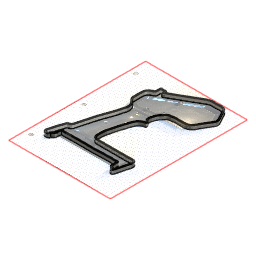
Emaxx MIrage Enclosure v0 (Autodesk Fusion 360 design; units mm, degrees)
Autodesk Fusion 360 part; units mm, degrees
sketch "Sketch2" plane through (0, 0, 0) normal (0, 0, 1) x (1, 0, 0)
  spline S0 degree 5 poles (-0.95, 3.75) (-0.9475, 3.7491) (-0.9413, 3.7486) (-0.9288, 3.7521) (-0.9057, 3.7644) (-0.869, 3.7885) (-0.8284, 3.8167) (-0.7876, 3.8442) (-0.7495, 3.8679) (-0.7146, 3.8869) (-0.6821, 3.9022) (-0.6502, 3.916) (-0.6169, 3.9306) (-0.5806, 3.948) (-0.5405, 3.9692) (-0.4968, 3.994) (-0.4504, 4.0216) (-0.4021, 4.0511) (-0.3533, 4.0811) (-0.3049, 4.1104) (-0.2575, 4.1384) (-0.2114, 4.1649) (-0.1663, 4.1901) (-0.1217, 4.2145) (-0.0769, 4.2387) (-0.0315, 4.2635) (0.0151, 4.2892) (0.0629, 4.316) (0.112, 4.3439) (0.1618, 4.3725) (0.2119, 4.4014) (0.2618, 4.43) (0.3108, 4.4579) (0.3585, 4.4847) (0.4045, 4.5102) (0.4488, 4.5344) (0.4913, 4.5578) (0.5322, 4.5804) (0.572, 4.6029) (0.6111, 4.6256) (0.6502, 4.649) (0.69, 4.6733) (0.7313, 4.6987) (0.7747, 4.7254) (0.8208, 4.7534) (0.8697, 4.7825) (0.9214, 4.8125) (0.9752, 4.8432) (1.0299, 4.8741) (1.0843, 4.9046) (1.137, 4.9344) (1.1865, 4.9628) (1.232, 4.9895) (1.2727, 5.0142) (1.3089, 5.0366) (1.3415, 5.0567) (1.3719, 5.0748) (1.4014, 5.0909) (1.4312, 5.1053) (1.4616, 5.1183) (1.4918, 5.1299) (1.5207, 5.1402) (1.5474, 5.1493) (1.5719, 5.1571) (1.5957, 5.1636) (1.6214, 5.1688) (1.6515, 5.1727) (1.6877, 5.1753) (1.7304, 5.1768) (1.7787, 5.1777) (1.831, 5.1781) (1.8853, 5.1784) (1.9398, 5.1788) (1.9928, 5.1796) (2.0435, 5.1807) (2.0916, 5.1822) (2.1375, 5.1838) (2.1815, 5.1854) (2.2245, 5.1869) (2.2669, 5.1882) (2.3091, 5.1891) (2.3512, 5.1898) (2.3932, 5.1902) (2.4348, 5.1903) (2.4757, 5.1899) (2.5154, 5.1887) (2.5536, 5.1862) (2.5898, 5.1817) (2.6236, 5.1747) (2.6548, 5.1647) (2.6834, 5.1517) (2.7093, 5.1358) (2.7329, 5.1173) (2.7545, 5.0963) (2.7746, 5.073) (2.7938, 5.047) (2.8124, 5.0181) (2.8309, 4.9862) (2.8494, 4.9516) (2.868, 4.9152) (2.8863, 4.8784) (2.9038, 4.8428) (2.9204, 4.8098) (2.9358, 4.7801) (2.9503, 4.7535) (2.9643, 4.7288) (2.9785, 4.7041) (2.9937, 4.6776) (3.0106, 4.6478) (3.0295, 4.6137) (3.0508, 4.5747) (3.0744, 4.5313) (3.0999, 4.4842) (3.1265, 4.4351) (3.1531, 4.3863) (3.1783, 4.3407) (3.2006, 4.3009) (3.2187, 4.2688) (3.2321, 4.245) (3.2409, 4.2282) (3.2464, 4.2145) (3.2505, 4.1992) (3.2546, 4.1789) (3.2598, 4.1536) (3.266, 4.1248) (3.2728, 4.0951) (3.2791, 4.0661) (3.2837, 4.0383) (3.2851, 4.0115) (3.2821, 3.985) (3.2741, 3.9576) (3.2612, 3.9283) (3.2437, 3.896) (3.2222, 3.8597) (3.1974, 3.8189) (3.1699, 3.7735) (3.1403, 3.7238) (3.109, 3.6706) (3.0764, 3.6146) (3.043, 3.5569) (3.0091, 3.4985) (2.9753, 3.4407) (2.942, 3.3841) (2.9097, 3.3298) (2.8789, 3.2782) (2.85, 3.2297) (2.8235, 3.1845) (2.7994, 3.1426) (2.7778, 3.1037) (2.7583, 3.0672) (2.7406, 3.0325) (2.7237, 2.9984) (2.7069, 2.9644) (2.6894, 2.9297) (2.6705, 2.8939) (2.6498, 2.8575) (2.627, 2.8209) (2.602, 2.785) (2.5747, 2.7507) (2.5451, 2.719) (2.5131, 2.6904) (2.4783, 2.6652) (2.4406, 2.6436) (2.3997, 2.6255) (2.3554, 2.6106) (2.3077, 2.5986) (2.2567, 2.5892) (2.2028, 2.582) (2.1464, 2.5769) (2.088, 2.5734) (2.0283, 2.5712) (1.9678, 2.5702) (1.907, 2.57) (1.8466, 2.5704) (1.7869, 2.5713) (1.7282, 2.5724) (1.6706, 2.5736) (1.6145, 2.5747) (1.5597, 2.5755) (1.5065, 2.5758) (1.4547, 2.5753) (1.4042, 2.5738) (1.355, 2.5709) (1.307, 2.5665) (1.2601, 2.5605) (1.2141, 2.5529) (1.1692, 2.5442) (1.1253, 2.5348) (1.0825, 2.5257) (1.041, 2.5175) (1.0009, 2.5106) (0.9622, 2.5051) (0.9252, 2.4999) (0.8897, 2.4934) (0.8558, 2.4834) (0.8232, 2.4678) (0.7918, 2.4453) (0.7614, 2.4157) (0.7315, 2.3802) (0.702, 2.3411) (0.6724, 2.3007) (0.6426, 2.2616) (0.6125, 2.2254) (0.5821, 2.1929) (0.5515, 2.1631) (0.5213, 2.1342) (0.4918, 2.104) (0.4634, 2.0703) (0.4367, 2.0318) (0.412, 1.9881) (0.3894, 1.9404) (0.3692, 1.8905) (0.3515, 1.8407) (0.336, 1.7932) (0.3227, 1.7498) (0.3113, 1.7112) (0.3014, 1.6772) (0.2925, 1.6462) (0.2843, 1.6167) (0.2765, 1.5869) (0.269, 1.556) (0.2617, 1.5236) (0.2552, 1.4898) (0.25, 1.4551) (0.2469, 1.4195) (0.2472, 1.3828) (0.2521, 1.3445) (0.2625, 1.3043) (0.2788, 1.2622) (0.3008, 1.2189) (0.3268, 1.1759) (0.3543, 1.1359) (0.3807, 1.1012) (0.4035, 1.074) (0.4216, 1.0551) (0.4356, 1.0436) (0.4477, 1.0366) (0.4596, 1.0305) (0.4686, 1.0229) (0.4685, 1.0131) (0.4592, 1.0035) (0.4471, 0.9978) (0.436, 0.9978) (0.4231, 1.0003) (0.4038, 1.0011) (0.3767, 0.9976) (0.3427, 0.9887) (0.3041, 0.9744) (0.2639, 0.9553) (0.2243, 0.9329) (0.1867, 0.9086) (0.1519, 0.8837) (0.1201, 0.8596) (0.0913, 0.8367) (0.065, 0.8149) (0.0406, 0.7931) (0.0175, 0.7696) (-0.0048, 0.7427) (-0.0267, 0.7112) (-0.0485, 0.6747) (-0.0701, 0.6339) (-0.0912, 0.5904) (-0.1115, 0.5459) (-0.1308, 0.5018) (-0.1487, 0.4596) (-0.1652, 0.4197) (-0.1804, 0.3815) (-0.1945, 0.3443) (-0.2078, 0.307) (-0.2206, 0.2687) (-0.233, 0.2294) (-0.2449, 0.1894) (-0.2564, 0.1499) (-0.2674, 0.112) (-0.2779, 0.0765) (-0.288, 0.0437) (-0.298, 0.0127) (-0.3085, -0.0181) (-0.3197, -0.0504) (-0.332, -0.0856) (-0.3451, -0.1237) (-0.3586, -0.1636) (-0.3717, -0.2034) (-0.3836, -0.2411) (-0.3939, -0.2749) (-0.4024, -0.3045) (-0.4097, -0.3309) (-0.4169, -0.3564) (-0.4249, -0.3836) (-0.4345, -0.4151) (-0.446, -0.4523) (-0.4593, -0.496) (-0.4738, -0.5462) (-0.4889, -0.6023) (-0.504, -0.663) (-0.5184, -0.7264) (-0.5319, -0.7901) (-0.5442, -0.8517) (-0.5555, -0.9084) (-0.566, -0.9582) (-0.5757, -0.9997) (-0.5851, -1.0326) (-0.5941, -1.0579) (-0.6028, -1.0786) (-0.6111, -1.0987) (-0.6189, -1.1217) (-0.6261, -1.1503) (-0.6329, -1.1849) (-0.6394, -1.225) (-0.6458, -1.269) (-0.6521, -1.3154) (-0.6584, -1.3628) (-0.6645, -1.4102) (-0.6701, -1.4572) (-0.6751, -1.5037) (-0.679, -1.5498) (-0.6819, -1.5956) (-0.6837, -1.6413) (-0.6844, -1.687) (-0.6843, -1.7325) (-0.6836, -1.7778) (-0.6824, -1.8227) (-0.6806, -1.8672) (-0.6778, -1.9109) (-0.6735, -1.9536) (-0.667, -1.9952) (-0.6574, -2.0354) (-0.644, -2.0738) (-0.6262, -2.1102) (-0.6039, -2.1443) (-0.577, -2.1756) (-0.5459, -2.2038) (-0.5112, -2.2287) (-0.4735, -2.2499) (-0.4341, -2.2674) (-0.3941, -2.281) (-0.3549, -2.291) (-0.3174, -2.2975) (-0.2827, -2.3011) (-0.2513, -2.3023) (-0.2231, -2.3019) (-0.1975, -2.3008) (-0.1733, -2.2996) (-0.1484, -2.2989) (-0.1198, -2.2988) (-0.0847, -2.2991) (-0.0408, -2.2998) (0.0131, -2.3004) (0.0766, -2.301) (0.1471, -2.3013) (0.2215, -2.3014) (0.2956, -2.3012) (0.3656, -2.3009) (0.428, -2.3005) (0.4805, -2.3001) (0.5223, -2.2998) (0.5549, -2.2997) (0.5819, -2.2997) (0.6078, -2.2998) (0.6374, -2.3001) (0.6744, -2.3003) (0.7211, -2.3006) (0.7787, -2.3009) (0.847, -2.3011) (0.9253, -2.3012) (1.012, -2.3011) (1.105, -2.3008) (1.2021, -2.3004) (1.3009, -2.2999) (1.3991, -2.2993) (1.4945, -2.2986) (1.5853, -2.2981) (1.6702, -2.2977) (1.748, -2.2975) (1.8179, -2.2976) (1.8797, -2.2981) (1.9336, -2.2988) (1.9802, -2.2997) (2.0208, -2.3007) (2.0572, -2.3015) (2.0915, -2.3019) (2.1261, -2.3016) (2.1628, -2.3005) (2.2031, -2.2985) (2.2474, -2.2961) (2.2952, -2.2935) (2.3455, -2.2914) (2.3967, -2.2901) (2.4466, -2.2897) (2.4931, -2.2903) (2.5337, -2.2911) (2.5664, -2.2915) (2.5903, -2.291) (2.6061, -2.2895) (2.6172, -2.2883) (2.6291, -2.2893) (2.6455, -2.2933) (2.6649, -2.2981) (2.6839, -2.3008) (2.7, -2.3016) (2.714, -2.3047) (2.728, -2.3149) (2.7429, -2.3326) (2.7584, -2.3539) (2.7733, -2.3746) (2.7863, -2.3924) (2.7959, -2.4095) (2.8013, -2.4294) (2.802, -2.4553) (2.7986, -2.4867) (2.792, -2.5219) (2.7834, -2.5581) (2.7739, -2.593) (2.7641, -2.6262) (2.7541, -2.6586) (2.7438, -2.6925) (2.7327, -2.7299) (2.7206, -2.7731) (2.7073, -2.8229) (2.6927, -2.8794) (2.6767, -2.9417) (2.6598, -3.0087) (2.642, -3.0785) (2.6237, -3.1493) (2.6056, -3.219) (2.5879, -3.2859) (2.5714, -3.3486) (2.5565, -3.4058) (2.5437, -3.4571) (2.5333, -3.502) (2.5253, -3.5406) (2.5194, -3.5732) (2.5146, -3.6005) (2.5099, -3.6233) (2.5037, -3.643) (2.4951, -3.6612) (2.4839, -3.68) (2.4709, -3.7011) (2.4573, -3.7246) (2.4445, -3.7472) (2.434, -3.7619) (2.4268, -3.762) (2.4227, -3.7469) (2.4205, -3.7222) (2.4191, -3.6951) (2.4184, -3.67) (2.4188, -3.6473) (2.4203, -3.6266) (2.4212, -3.6077) (2.4171, -3.5929) (2.4041, -3.5847) (2.3819, -3.5833) (2.3542, -3.5865) (2.3257, -3.5909) (2.3001, -3.5933) (2.2787, -3.5913) (2.2609, -3.5831) (2.2459, -3.5674) (2.2332, -3.5432) (2.2225, -3.5098) (2.2141, -3.4673) (2.2079, -3.4165) (2.2037, -3.3595) (2.2009, -3.2998) (2.1987, -3.2412) (2.1965, -3.1875) (2.1939, -3.1416) (2.1907, -3.1053) (2.1877, -3.0784) (2.1863, -3.0579) (2.1879, -3.0395) (2.1922, -3.0196) (2.1952, -2.9981) (2.1906, -2.9775) (2.1729, -2.9613) (2.1414, -2.9514) (2.1005, -2.9473) (2.0571, -2.9474) (2.0178, -2.9495) (1.987, -2.9514) (1.9639, -2.9522) (1.9434, -2.9515) (1.9189, -2.9499) (1.8844, -2.9478) (1.8365, -2.9456) (1.7739, -2.9436) (1.697, -2.9422) (1.6078, -2.9414) (1.5091, -2.9414) (1.4044, -2.9422) (1.2973, -2.9438) (1.1916, -2.9461) (1.0903, -2.9491) (0.9957, -2.9526) (0.9088, -2.9565) (0.8294, -2.9606) (0.7564, -2.9648) (0.6878, -2.9689) (0.6214, -2.9727) (0.5545, -2.9762) (0.4845, -2.9791) (0.409, -2.9815) (0.3258, -2.9832) (0.2336, -2.9843) (0.1317, -2.9847) (0.0203, -2.9845) (-0.1, -2.9839) (-0.228, -2.9829) (-0.3621, -2.9817) (-0.5004, -2.9805) (-0.6409, -2.9793) (-0.7812, -2.9783) (-0.9193, -2.9777) (-1.0531, -2.9775) (-1.1806, -2.9779) (-1.3005, -2.9788) (-1.4115, -2.9804) (-1.513, -2.9825) (-1.605, -2.9851) (-1.6882, -2.988) (-1.7639, -2.9911) (-1.8336, -2.994) (-1.8992, -2.9965) (-1.9623, -2.9986) (-2.0243, -2.9999) (-2.0862, -3.0005) (-2.1483, -3.0002) (-2.21, -2.9992) (-2.2697, -2.9977) (-2.3252, -2.9961) (-2.3741, -2.995) (-2.4146, -2.9952) (-2.4455, -2.9977) (-2.4674, -3.004) (-2.4824, -3.0159) (-2.4942, -3.0351) (-2.5057, -3.0628) (-2.5184, -3.0989) (-2.5312, -3.1418) (-2.5423, -3.1893) (-2.5496, -3.2388) (-2.5516, -3.2878) (-2.5484, -3.3344) (-2.5427, -3.3775) (-2.5391, -3.417) (-2.5424, -3.4535) (-2.5569, -3.4871) (-2.5845, -3.5182) (-2.6236, -3.546) (-2.6692, -3.5692) (-2.715, -3.5867) (-2.7546, -3.5981) (-2.7831, -3.6044) (-2.7991, -3.6085) (-2.8055, -3.616) (-2.8072, -3.6317) (-2.8077, -3.6559) (-2.8087, -3.685) (-2.8102, -3.7139) (-2.8116, -3.7385) (-2.8114, -3.7576) (-2.8096, -3.772) (-2.8089, -3.7827) (-2.8163, -3.7905) (-2.8371, -3.7957) (-2.8698, -3.7986) (-2.9085, -3.7994) (-2.946, -3.7982) (-2.9762, -3.7947) (-2.9978, -3.7883) (-3.0132, -3.7783) (-3.0259, -3.7642) (-3.0382, -3.7454) (-3.0499, -3.722) (-3.0598, -3.6944) (-3.0664, -3.6636) (-3.0689, -3.6309) (-3.0672, -3.5981) (-3.0615, -3.5667) (-3.0526, -3.5375) (-3.0414, -3.5102) (-3.029, -3.4838) (-3.0165, -3.4566) (-3.0046, -3.4272) (-2.9937, -3.3948) (-2.9837, -3.3593) (-2.9744, -3.3214) (-2.9652, -3.2818) (-2.9557, -3.2414) (-2.9456, -3.201) (-2.935, -3.1609) (-2.924, -3.1212) (-2.9129, -3.0819) (-2.9018, -3.0432) (-2.8912, -3.0051) (-2.8811, -2.9678) (-2.8718, -2.9316) (-2.863, -2.8969) (-2.8545, -2.8636) (-2.8459, -2.8317) (-2.8365, -2.8009) (-2.8256, -2.7708) (-2.8129, -2.7407) (-2.7985, -2.7105) (-2.7832, -2.6802) (-2.7687, -2.6503) (-2.7563, -2.6209) (-2.7471, -2.5923) (-2.7411, -2.5642) (-2.7373, -2.5356) (-2.7337, -2.5058) (-2.7284, -2.4744) (-2.7203, -2.4421) (-2.7087, -2.411) (-2.6938, -2.3834) (-2.676, -2.3615) (-2.6559, -2.3462) (-2.6333, -2.3362) (-2.6085, -2.3294) (-2.5813, -2.3227) (-2.5521, -2.314) (-2.5217, -2.302) (-2.4912, -2.2863) (-2.4615, -2.2667) (-2.4337, -2.2435) (-2.4086, -2.217) (-2.3867, -2.1873) (-2.3684, -2.1548) (-2.3534, -2.1198) (-2.3414, -2.0825) (-2.3316, -2.0433) (-2.323, -2.0027) (-2.3144, -1.961) (-2.3049, -1.9186) (-2.294, -1.8759) (-2.2816, -1.8329) (-2.2679, -1.7898) (-2.2538, -1.7466) (-2.2399, -1.7034) (-2.227, -1.6602) (-2.2155, -1.6171) (-2.2055, -1.5743) (-2.1966, -1.5322) (-2.1881, -1.491) (-2.1794, -1.4507) (-2.1699, -1.4113) (-2.1592, -1.3723) (-2.1471, -1.3328) (-2.1339, -1.292) (-2.1199, -1.2489) (-2.1056, -1.2029) (-2.0912, -1.1537) (-2.0774, -1.1019) (-2.0641, -1.0488) (-2.0516, -0.9961) (-2.0398, -0.9457) (-2.0287, -0.8991) (-2.0183, -0.8574) (-2.0082, -0.8208) (-1.9984, -0.7883) (-1.9887, -0.7578) (-1.9789, -0.7271) (-1.9687, -0.694) (-1.9579, -0.657) (-1.9463, -0.6154) (-1.9337, -0.5694) (-1.9199, -0.5196) (-1.9049, -0.467) (-1.8885, -0.4129) (-1.871, -0.3581) (-1.8523, -0.3036) (-1.8329, -0.2497) (-1.8131, -0.1969) (-1.7932, -0.1451) (-1.7736, -0.0945) (-1.7545, -0.0451) (-1.7363, 0.0034) (-1.7189, 0.0507) (-1.7023, 0.0971) (-1.6866, 0.1423) (-1.6714, 0.1866) (-1.6568, 0.23) (-1.6424, 0.2726) (-1.628, 0.3148) (-1.6135, 0.3569) (-1.5988, 0.3995) (-1.5837, 0.443) (-1.5683, 0.4877) (-1.5526, 0.5339) (-1.5369, 0.5816) (-1.5213, 0.6308) (-1.5062, 0.681) (-1.4919, 0.7318) (-1.4786, 0.7829) (-1.4663, 0.8335) (-1.455, 0.8832) (-1.4444, 0.9312) (-1.4341, 0.9772) (-1.4235, 1.0208) (-1.4124, 1.0616) (-1.4004, 1.0998) (-1.3877, 1.1358) (-1.3748, 1.1701) (-1.3623, 1.2038) (-1.3511, 1.2377) (-1.3418, 1.2728) (-1.335, 1.3096) (-1.3308, 1.3481) (-1.3291, 1.3884) (-1.3297, 1.4299) (-1.3323, 1.4723) (-1.3368, 1.5152) (-1.3434, 1.5582) (-1.3525, 1.6013) (-1.3643, 1.6444) (-1.3792, 1.6872) (-1.3974, 1.7296) (-1.4188, 1.7711) (-1.4428, 1.8112) (-1.4689, 1.8491) (-1.4961, 1.8842) (-1.5236, 1.9161) (-1.551, 1.9446) (-1.5778, 1.9701) (-1.6041, 1.9935) (-1.6302, 2.016) (-1.6561, 2.0386) (-1.6818, 2.0623) (-1.7069, 2.0876) (-1.7303, 2.1143) (-1.751, 2.142) (-1.7681, 2.1705) (-1.781, 2.1998) (-1.7898, 2.2305) (-1.795, 2.2636) (-1.7976, 2.2999) (-1.7984, 2.3404) (-1.7983, 2.3856) (-1.798, 2.4353) (-1.7978, 2.4889) (-1.7979, 2.5453) (-1.7984, 2.6036) (-1.7993, 2.6625) (-1.8004, 2.7209) (-1.8016, 2.7779) (-1.8027, 2.8327) (-1.8034, 2.8851) (-1.8034, 2.9347) (-1.8026, 2.9815) (-1.8005, 3.0257) (-1.7968, 3.0672) (-1.7912, 3.1064) (-1.7834, 3.1435) (-1.7729, 3.1788) (-1.7596, 3.2124) (-1.7432, 3.2445) (-1.7236, 3.2753) (-1.7008, 3.3046) (-1.675, 3.3325) (-1.6463, 3.3588) (-1.6151, 3.3836) (-1.5821, 3.4067) (-1.5478, 3.4282) (-1.513, 3.4483) (-1.4782, 3.467) (-1.4442, 3.4846) (-1.4114, 3.5015) (-1.3801, 3.5178) (-1.3507, 3.534) (-1.3238, 3.55) (-1.3004, 3.5656) (-1.2818, 3.5802) (-1.2693, 3.5933) (-1.2631, 3.6054) (-1.2618, 3.6189) (-1.2626, 3.6373) (-1.2631, 3.6633) (-1.2626, 3.698) (-1.2616, 3.7406) (-1.261, 3.7892) (-1.2616, 3.8407) (-1.2639, 3.8914) (-1.2672, 3.937) (-1.2698, 3.9733) (-1.2701, 3.9974) (-1.2665, 4.0079) (-1.2586, 4.0066) (-1.2472, 3.998) (-1.233, 3.9874) (-1.2159, 3.9784) (-1.1957, 3.973) (-1.1731, 3.9708) (-1.1494, 3.9697) (-1.1256, 3.9675) (-1.102, 3.9639) (-1.0772, 3.9617) (-1.0496, 3.9646) (-1.019, 3.9745) (-0.9883, 3.989) (-0.963, 4.0009) (-0.9481, 4.0034) (-0.9453, 3.9939) (-0.9493, 3.9789) (-0.9524, 3.9668) (-0.9517, 3.9575) (-0.9486, 3.9442) (-0.9457, 3.9222) (-0.9449, 3.8916) (-0.9473, 3.855) (-0.9527, 3.817) (-0.9584, 3.7831) (-0.9595, 3.7632) (-0.9566, 3.7542) (-0.9525, 3.7509) (-0.95, 3.75) knots 0 0 0 0 0 0 0.00123457 0.00246914 0.0037037 0.00493827 0.00617284 0.00740741 0.00864198 0.00987654 0.01111111 0.01234568 0.01358025 0.01481481 0.01604938 0.01728395 0.01851852 0.01975309 0.02098765 0.02222222 0.02345679 0.02469136 0.02592593 0.02716049 0.02839506 0.02962963 0.0308642 0.03209877 0.03333333 0.0345679 0.03580247 0.03703704 0.0382716 0.03950617 0.04074074 0.04197531 0.04320988 0.04444444 0.04567901 0.04691358 0.04814815 0.04938272 0.05061728 0.05185185 0.05308642 0.05432099 0.05555556 0.05679012 0.05802469 0.05925926 0.06049383 0.0617284 0.06296296 0.06419753 0.0654321 0.06666667 0.06790123 0.0691358 0.07037037 0.07160494 0.07283951 0.07407407 0.07530864 0.07654321 0.07777778 0.07901235 0.08024691 0.08148148 0.08271605 0.08395062 0.08518519 0.08641975 0.08765432 0.08888889 0.09012346 0.09135802 0.09259259 0.09382716 0.09506173 0.0962963 0.09753086 0.09876543 0.1 0.10123457 0.10246914 0.1037037 0.10493827 0.10617284 0.10740741 0.10864198 0.10987654 0.11111111 0.11234568 0.11358025 0.11481481 0.11604938 0.11728395 0.11851852 0.11975309 0.12098765 0.12222222 0.12345679 0.12469136 0.12592593 0.12716049 0.12839506 0.12962963 0.1308642 0.13209877 0.13333333 0.1345679 0.13580247 0.13703704 0.1382716 0.13950617 0.14074074 0.14197531 0.14320988 0.14444444 0.14567901 0.14691358 0.14814815 0.14938272 0.15061728 0.15185185 0.15308642 0.15432099 0.15555556 0.15679012 0.15802469 0.15925926 0.16049383 0.1617284 0.16296296 0.16419753 0.1654321 0.16666667 0.16790123 0.1691358 0.17037037 0.17160494 0.17283951 0.17407407 0.17530864 0.17654321 0.17777778 0.17901235 0.18024691 0.18148148 0.18271605 0.18395062 0.18518519 0.18641975 0.18765432 0.18888889 0.19012346 0.19135802 0.19259259 0.19382716 0.19506173 0.1962963 0.19753086 0.19876543 0.2 0.20123457 0.20246914 0.2037037 0.20493827 0.20617284 0.20740741 0.20864198 0.20987654 0.21111111 0.21234568 0.21358025 0.21481481 0.21604938 0.21728395 0.21851852 0.21975309 0.22098765 0.22222222 0.22345679 0.22469136 0.22592593 0.22716049 0.22839506 0.22962963 0.2308642 0.23209877 0.23333333 0.2345679 0.23580247 0.23703704 0.2382716 0.23950617 0.24074074 0.24197531 0.24320988 0.24444444 0.24567901 0.24691358 0.24814815 0.24938272 0.25061728 0.25185185 0.25308642 0.25432099 0.25555556 0.25679012 0.25802469 0.25925926 0.26049383 0.2617284 0.26296296 0.26419753 0.2654321 0.26666667 0.26790123 0.2691358 0.27037037 0.27160494 0.27283951 0.27407407 0.27530864 0.27654321 0.27777778 0.27901235 0.28024691 0.28148148 0.28271605 0.28395062 0.28518519 0.28641975 0.28765432 0.28888889 0.29012346 0.29135802 0.29259259 0.29382716 0.29506173 0.2962963 0.29753086 0.29876543 0.3 0.30123457 0.30246914 0.3037037 0.30493827 0.30617284 0.30740741 0.30864198 0.30987654 0.31111111 0.31234568 0.31358025 0.31481481 0.31604938 0.31728395 0.31851852 0.31975309 0.32098765 0.32222222 0.32345679 0.32469136 0.32592593 0.32716049 0.32839506 0.32962963 0.3308642 0.33209877 0.33333333 0.3345679 0.33580247 0.33703704 0.3382716 0.33950617 0.34074074 0.34197531 0.34320988 0.34444444 0.34567901 0.34691358 0.34814815 0.34938272 0.35061728 0.35185185 0.35308642 0.35432099 0.35555556 0.35679012 0.35802469 0.35925926 0.36049383 0.3617284 0.36296296 0.36419753 0.3654321 0.36666667 0.36790123 0.3691358 0.37037037 0.37160494 0.37283951 0.37407407 0.37530864 0.37654321 0.37777778 0.37901235 0.38024691 0.38148148 0.38271605 0.38395062 0.38518519 0.38641975 0.38765432 0.38888889 0.39012346 0.39135802 0.39259259 0.39382716 0.39506173 0.3962963 0.39753086 0.39876543 0.4 0.40123457 0.40246914 0.4037037 0.40493827 0.40617284 0.40740741 0.40864198 0.40987654 0.41111111 0.41234568 0.41358025 0.41481481 0.41604938 0.41728395 0.41851852 0.41975309 0.42098765 0.42222222 0.42345679 0.42469136 0.42592593 0.42716049 0.42839506 0.42962963 0.4308642 0.43209877 0.43333333 0.4345679 0.43580247 0.43703704 0.4382716 0.43950617 0.44074074 0.44197531 0.44320988 0.44444444 0.44567901 0.44691358 0.44814815 0.44938272 0.45061728 0.45185185 0.45308642 0.45432099 0.45555556 0.45679012 0.45802469 0.45925926 0.46049383 0.4617284 0.46296296 0.46419753 0.4654321 0.46666667 0.46790123 0.4691358 0.47037037 0.47160494 0.47283951 0.47407407 0.47530864 0.47654321 0.47777778 0.47901235 0.48024691 0.48148148 0.48271605 0.48395062 0.48518519 0.48641975 0.48765432 0.48888889 0.49012346 0.49135802 0.49259259 0.49382716 0.49506173 0.4962963 0.49753086 0.49876543 0.5 0.50123457 0.50246914 0.5037037 0.50493827 0.50617284 0.50740741 0.50864198 0.50987654 0.51111111 0.51234568 0.51358025 0.51481481 0.51604938 0.51728395 0.51851852 0.51975309 0.52098765 0.52222222 0.52345679 0.52469136 0.52592593 0.52716049 0.52839506 0.52962963 0.5308642 0.53209877 0.53333333 0.5345679 0.53580247 0.53703704 0.5382716 0.53950617 0.54074074 0.54197531 0.54320988 0.54444444 0.54567901 0.54691358 0.54814815 0.54938272 0.55061728 0.55185185 0.55308642 0.55432099 0.55555556 0.55679012 0.55802469 0.55925926 0.56049383 0.5617284 0.56296296 0.56419753 0.5654321 0.56666667 0.56790123 0.5691358 0.57037037 0.57160494 0.57283951 0.57407407 0.57530864 0.57654321 0.57777778 0.57901235 0.58024691 0.58148148 0.58271605 0.58395062 0.58518519 0.58641975 0.58765432 0.58888889 0.59012346 0.59135802 0.59259259 0.59382716 0.59506173 0.5962963 0.59753086 0.59876543 0.6 0.60123457 0.60246914 0.6037037 0.60493827 0.60617284 0.60740741 0.60864198 0.60987654 0.61111111 0.61234568 0.61358025 0.61481481 0.61604938 0.61728395 0.61851852 0.61975309 0.62098765 0.62222222 0.62345679 0.62469136 0.62592593 0.62716049 0.62839506 0.62962963 0.6308642 0.63209877 0.63333333 0.6345679 0.63580247 0.63703704 0.6382716 0.63950617 0.64074074 0.64197531 0.64320988 0.64444444 0.64567901 0.64691358 0.64814815 0.64938272 0.65061728 0.65185185 0.65308642 0.65432099 0.65555556 0.65679012 0.65802469 0.65925926 0.66049383 0.6617284 0.66296296 0.66419753 0.6654321 0.66666667 0.66790123 0.6691358 0.67037037 0.67160494 0.67283951 0.67407407 0.67530864 0.67654321 0.67777778 0.67901235 0.68024691 0.68148148 0.68271605 0.68395062 0.68518519 0.68641975 0.68765432 0.68888889 0.69012346 0.69135802 0.69259259 0.69382716 0.69506173 0.6962963 0.69753086 0.69876543 0.7 0.70123457 0.70246914 0.7037037 0.70493827 0.70617284 0.70740741 0.70864198 0.70987654 0.71111111 0.71234568 0.71358025 0.71481481 0.71604938 0.71728395 0.71851852 0.71975309 0.72098765 0.72222222 0.72345679 0.72469136 0.72592593 0.72716049 0.72839506 0.72962963 0.7308642 0.73209877 0.73333333 0.7345679 0.73580247 0.73703704 0.7382716 0.73950617 0.74074074 0.74197531 0.74320988 0.74444444 0.74567901 0.74691358 0.74814815 0.74938272 0.75061728 0.75185185 0.75308642 0.75432099 0.75555556 0.75679012 0.75802469 0.75925926 0.76049383 0.7617284 0.76296296 0.76419753 0.7654321 0.76666667 0.76790123 0.7691358 0.77037037 0.77160494 0.77283951 0.77407407 0.77530864 0.77654321 0.77777778 0.77901235 0.78024691 0.78148148 0.78271605 0.78395062 0.78518519 0.78641975 0.78765432 0.78888889 0.79012346 0.79135802 0.79259259 0.79382716 0.79506173 0.7962963 0.79753086 0.79876543 0.8 0.80123457 0.80246914 0.8037037 0.80493827 0.80617284 0.80740741 0.80864198 0.80987654 0.81111111 0.81234568 0.81358025 0.81481481 0.81604938 0.81728395 0.81851852 0.81975309 0.82098765 0.82222222 0.82345679 0.82469136 0.82592593 0.82716049 0.82839506 0.82962963 0.8308642 0.83209877 0.83333333 0.8345679 0.83580247 0.83703704 0.8382716 0.83950617 0.84074074 0.84197531 0.84320988 0.84444444 0.84567901 0.84691358 0.84814815 0.84938272 0.85061728 0.85185185 0.85308642 0.85432099 0.85555556 0.85679012 0.85802469 0.85925926 0.86049383 0.8617284 0.86296296 0.86419753 0.8654321 0.86666667 0.86790123 0.8691358 0.87037037 0.87160494 0.87283951 0.87407407 0.87530864 0.87654321 0.87777778 0.87901235 0.88024691 0.88148148 0.88271605 0.88395062 0.88518519 0.88641975 0.88765432 0.88888889 0.89012346 0.89135802 0.89259259 0.89382716 0.89506173 0.8962963 0.89753086 0.89876543 0.9 0.90123457 0.90246914 0.9037037 0.90493827 0.90617284 0.90740741 0.90864198 0.90987654 0.91111111 0.91234568 0.91358025 0.91481481 0.91604938 0.91728395 0.91851852 0.91975309 0.92098765 0.92222222 0.92345679 0.92469136 0.92592593 0.92716049 0.92839506 0.92962963 0.9308642 0.93209877 0.93333333 0.9345679 0.93580247 0.93703704 0.9382716 0.93950617 0.94074074 0.94197531 0.94320988 0.94444444 0.94567901 0.94691358 0.94814815 0.94938272 0.95061728 0.95185185 0.95308642 0.95432099 0.95555556 0.95679012 0.95802469 0.95925926 0.96049383 0.9617284 0.96296296 0.96419753 0.9654321 0.96666667 0.96790123 0.9691358 0.97037037 0.97160494 0.97283951 0.97407407 0.97530864 0.97654321 0.97777778 0.97901235 0.98024691 0.98148148 0.98271605 0.98395062 0.98518519 0.98641975 0.98765432 0.98888889 0.99012346 0.99135802 0.99259259 0.99382716 0.99506173 0.9962963 0.99753086 0.99876543 1 1 1 1 1 1
  spline S1 degree 3 poles (-1.1781, 4.0748) (-1.1778, 4.0746) (-1.1779, 4.0746) (-1.1781, 4.0748) knots 0.970853 0.970853 0.970853 0.970853 0.971274 0.971274 0.971274 0.971274
  spline S2 degree 3 poles (-0.8442, 3.9291) (-0.831, 3.9376) (-0.8196, 3.9447) (-0.8076, 3.9518) (-0.6925, 4.0201) (-0.6238, 4.0366) (-0.494, 4.1151) (-0.2507, 4.2622) (-0.0052, 4.3964) (0.2498, 4.5409) (0.4771, 4.6697) (0.6102, 4.7503) (0.8547, 4.8921) (1.0195, 4.9876) (1.1869, 5.0829) (1.2903, 5.1452) (1.3922, 5.2066) (1.4819, 5.2438) (1.5826, 5.2652) (1.7143, 5.2931) (1.9719, 5.2803) (2.1505, 5.2867) (2.3228, 5.293) (2.4851, 5.3166) (2.6506, 5.2725) (2.8553, 5.2181) (2.9472, 4.9806) (3.0181, 4.8439) (3.063, 4.7576) (3.1018, 4.6958) (3.1788, 4.5535) (3.238, 4.4442) (3.3, 4.3371) (3.3276, 4.283) (3.3619, 4.2161) (3.3764, 4.1556) (3.3855, 4.041) (3.398, 3.8843) (3.2626, 3.7314) (3.1297, 3.5024) (3.0163, 3.3067) (2.9061, 3.1292) (2.8466, 3.0146) (2.7855, 2.8971) (2.7326, 2.7484) (2.5954, 2.6273) (2.3571, 2.417) (1.9073, 2.4684) (1.5838, 2.4727) (1.3679, 2.4756) (1.2067, 2.4419) (1.0363, 2.4129) (0.9025, 2.3902) (0.8746, 2.4006) (0.7847, 2.2804) (0.7152, 2.1875) (0.6188, 2.0932) (0.5622, 2.0279) (0.482, 1.9353) (0.4248, 1.7364) (0.3949, 1.6315) (0.3655, 1.5286) (0.3307, 1.4414) (0.3586, 1.3443) (0.3758, 1.2844) (0.444, 1.1836) (0.4782, 1.1449) (0.4967, 1.1238) (0.4848, 1.1335) (0.5024, 1.1234) (0.513, 1.1174) (0.5634, 1.1007) (0.5694, 1.027) (0.5768, 0.9373) (0.5186, 0.9132) (0.4769, 0.9011) (0.425, 0.8861) (0.4162, 0.8984) (0.4082, 0.8979) (0.385, 0.8963) (0.2309, 0.8181) (0.1538, 0.7553) (0.088, 0.7017) (0.0554, 0.6595) (0.0045, 0.5526) (-0.0868, 0.3608) (-0.1391, 0.1779) (-0.1878, 0.0214) (-0.2297, -0.1128) (-0.2857, -0.2691) (-0.3163, -0.3767) (-0.3389, -0.4565) (-0.3867, -0.5992) (-0.4254, -0.7818) (-0.458, -0.936) (-0.4874, -1.0672) (-0.508, -1.1175) (-0.5249, -1.1586) (-0.5324, -1.1983) (-0.5451, -1.2891) (-0.5748, -1.5008) (-0.5919, -1.7342) (-0.5741, -1.9164) (-0.5609, -2.0511) (-0.509, -2.1258) (-0.3996, -2.1699) (-0.2973, -2.2111) (-0.2319, -2.1966) (-0.1261, -2.1965) (-0.0505, -2.1964) (0.1093, -2.1993) (0.2788, -2.1988) (0.439, -2.1984) (0.5332, -2.1971) (0.5937, -2.1974) (0.6617, -2.1977) (0.7841, -2.199) (1.0062, -2.1987) (1.3039, -2.1982) (1.6792, -2.1938) (1.8761, -2.1957) (2.079, -2.1977) (2.1306, -2.1983) (2.3057, -2.1907) (2.4079, -2.1862) (2.5287, -2.1895) (2.5715, -2.1889) (2.5974, -2.1885) (2.6142, -2.1834) (2.6474, -2.1891) (2.6891, -2.1963) (2.6669, -2.1838) (2.7389, -2.2065) (2.8053, -2.2274) (2.8328, -2.282) (2.8534, -2.3106) (2.8811, -2.3489) (2.9098, -2.4465) (2.8956, -2.5234) (2.8707, -2.6588) (2.8364, -2.7306) (2.7837, -2.9367) (2.7335, -3.1334) (2.661, -3.3989) (2.6336, -3.524) (2.6155, -3.6062) (2.6097, -3.6653) (2.5806, -3.7173) (2.5623, -3.7498) (2.5541, -3.7674) (2.5268, -3.8072) (2.5187, -3.8191) (2.5229, -3.8484) (2.4486, -3.861) (2.3957, -3.87) (2.3434, -3.8205) (2.3336, -3.7996) (2.3055, -3.7398) (2.3186, -3.7331) (2.3175, -3.7101) (2.3172, -3.7047) (2.317, -3.7) (2.3168, -3.6941) knots 0.00616262 0.00616262 0.00616262 0.00616262 0.00723627 0.00723627 0.00723627 0.01751679 0.01751679 0.01751679 0.03677766 0.03677766 0.03677766 0.05394591 0.05394591 0.05394591 0.0655192 0.0655192 0.0655192 0.07691737 0.07691737 0.07691737 0.09183359 0.09183359 0.09183359 0.10622417 0.10622417 0.10622417 0.12401706 0.12401706 0.12401706 0.13525578 0.13525578 0.13525578 0.14388411 0.14388411 0.14388411 0.15457935 0.15457935 0.15457935 0.1691993 0.1691993 0.1691993 0.1816861 0.1816861 0.1816861 0.19448952 0.19448952 0.19448952 0.21671489 0.21671489 0.21671489 0.23154272 0.23154272 0.23154272 0.24318105 0.24318105 0.24318105 0.25216346 0.25216346 0.25216346 0.26491111 0.26491111 0.26491111 0.27740929 0.27740929 0.27740929 0.28512377 0.28512377 0.28512377 0.28932444 0.28932444 0.28932444 0.29185971 0.29185971 0.29185971 0.29494795 0.29494795 0.29494795 0.29878542 0.29878542 0.29878542 0.30999878 0.30999878 0.30999878 0.31957073 0.31957073 0.31957073 0.33674276 0.33674276 0.33674276 0.35146989 0.35146989 0.35146989 0.36239404 0.36239404 0.36239404 0.3716135 0.3716135 0.3716135 0.37915533 0.37915533 0.37915533 0.39674759 0.39674759 0.39674759 0.409754 0.409754 0.409754 0.42191304 0.42191304 0.42191304 0.43059904 0.43059904 0.43059904 0.43880725 0.43880725 0.43880725 0.44804944 0.44804944 0.44804944 0.46043699 0.46043699 0.46043699 0.47319866 0.47319866 0.47319866 0.48065115 0.48065115 0.48065115 0.48517241 0.48517241 0.48517241 0.49084682 0.49084682 0.49084682 0.49608592 0.49608592 0.49608592 0.50309626 0.50309626 0.50309626 0.51543546 0.51543546 0.51543546 0.52720795 0.52720795 0.52720795 0.53495085 0.53495085 0.53495085 0.53980081 0.53980081 0.53980081 0.54125044 0.54125044 0.54125044 0.54228047 0.54228047 0.54228047 0.54523202 0.54523202 0.54523202 0.54591987 0.54591987 0.54591987 0.54591987
  spline S3 degree 3 poles (2.3168, -3.6941) (2.2745, -3.6967) (2.2158, -3.6835) (2.1787, -3.6439) (2.0885, -3.5476) (2.1027, -3.4054) (2.0973, -3.2692) (2.093, -3.1611) (2.0827, -3.1042) (2.0848, -3.0503) knots 0.557546 0.557546 0.557546 0.557546 0.561139 0.561139 0.561139 0.569876 0.569876 0.569876 0.576809 0.576809 0.576809 0.576809
  spline S4 degree 3 poles (2.0848, -3.0503) (2.0519, -3.0495) (2.0083, -3.0532) (1.9769, -3.0541) (1.914, -3.0557) (1.8638, -3.0467) (1.6811, -3.0446) (1.4518, -3.0419) (1.104, -3.0493) (0.8847, -3.0604) (0.6142, -3.074) (0.4496, -3.0875) (0.0692, -3.0869) (-0.3358, -3.0864) (-0.9379, -3.0766) (-1.3397, -3.0819) (-1.6837, -3.0865) (-1.8681, -3.1012) (-2.0636, -3.1026) (-2.1945, -3.1034) (-2.3414, -3.0961) (-2.4037, -3.0979) (-2.4056, -3.098) (-2.4075, -3.098) (-2.4091, -3.0981) knots 0.585558 0.585558 0.585558 0.585558 0.589601 0.589601 0.589601 0.597702 0.597702 0.597702 0.607877 0.607877 0.607877 0.620432 0.620432 0.620432 0.633798 0.633798 0.633798 0.645242 0.645242 0.645242 0.6529 0.6529 0.6529 0.653133 0.653133 0.653133 0.653133
  spline S5 degree 3 poles (-2.4091, -3.0981) (-2.4214, -3.1296) (-2.4451, -3.2085) (-2.4476, -3.267) (-2.4501, -3.3253) (-2.4183, -3.3842) (-2.4479, -3.4849) (-2.4783, -3.5888) (-2.5915, -3.6504) (-2.6726, -3.6794) (-2.6846, -3.6836) (-2.6951, -3.6871) (-2.7065, -3.6904) knots 0.659095 0.659095 0.659095 0.659095 0.664802 0.664802 0.664802 0.670488 0.670488 0.670488 0.676356 0.676356 0.676356 0.677225 0.677225 0.677225 0.677225
  spline S6 degree 3 poles (-2.7065, -3.6904) (-2.7075, -3.7118) (-2.7086, -3.7294) (-2.7088, -3.7401) (-2.7092, -3.754) (-2.7005, -3.734) (-2.7086, -3.7923) (-2.7139, -3.8316) (-2.7697, -3.8825) (-2.7978, -3.8906) (-2.8734, -3.9124) (-2.9313, -3.908) (-2.999, -3.8934) (-3.0669, -3.8787) (-3.1172, -3.8219) (-3.1422, -3.7646) (-3.1861, -3.6638) (-3.1515, -3.5055) (-3.1189, -3.434) (-3.0881, -3.3666) (-3.0713, -3.2788) (-3.0431, -3.1696) (-2.9974, -2.9927) (-2.9722, -2.8478) (-2.9073, -2.7019) (-2.8724, -2.6232) (-2.8479, -2.5879) (-2.8396, -2.5276) (-2.8313, -2.4674) (-2.8148, -2.3352) (-2.7219, -2.2689) (-2.6194, -2.1957) (-2.5669, -2.2182) (-2.5186, -2.1801) (-2.4517, -2.1275) (-2.438, -2.022) (-2.3959, -1.8617) (-2.32, -1.5731) (-2.2498, -1.3694) (-2.1691, -1.0461) (-2.1322, -0.8985) (-2.1026, -0.7798) (-2.0746, -0.6898) (-2.0289, -0.543) (-1.9312, -0.2219) (-1.8459, 0.003) (-1.7532, 0.2475) (-1.6856, 0.4393) (-1.6116, 0.6864) (-1.552, 0.8854) (-1.5063, 1.105) (-1.4613, 1.2321) (-1.4282, 1.3254) (-1.424, 1.4208) (-1.4438, 1.5344) (-1.4692, 1.6801) (-1.5635, 1.8192) (-1.6578, 1.904) (-1.7444, 1.982) (-1.8799, 2.1019) (-1.8965, 2.2564) (-1.9121, 2.4022) (-1.9004, 2.5956) (-1.9041, 2.7825) (-1.909, 3.029) (-1.9046, 3.2315) (-1.7665, 3.3837) (-1.6617, 3.4993) (-1.5077, 3.5646) (-1.4171, 3.6145) (-1.396, 3.6261) (-1.3775, 3.6373) (-1.3651, 3.6459) knots 0.68523181 0.68523181 0.68523181 0.68523181 0.68768508 0.68768508 0.68768508 0.69090518 0.69090518 0.69090518 0.6930744 0.6930744 0.6930744 0.69892381 0.69892381 0.69892381 0.70480591 0.70480591 0.70480591 0.71513992 0.71513992 0.71513992 0.72487251 0.72487251 0.72487251 0.74062751 0.74062751 0.74062751 0.74911807 0.74911807 0.74911807 0.75760153 0.75760153 0.75760153 0.76696121 0.76696121 0.76696121 0.77990358 0.77990358 0.77990358 0.80318753 0.80318753 0.80318753 0.81382154 0.81382154 0.81382154 0.83116808 0.83116808 0.83116808 0.85002594 0.85002594 0.85002594 0.86521338 0.86521338 0.86521338 0.87636452 0.87636452 0.87636452 0.89066357 0.89066357 0.89066357 0.90380639 0.90380639 0.90380639 0.91620826 0.91620826 0.91620826 0.93256382 0.93256382 0.93256382 0.94497795 0.94497795 0.94497795 0.94785846 0.94785846 0.94785846 0.94785846
  spline S7 degree 3 poles (-1.3651, 3.6459) (-1.3651, 3.6474) (-1.3651, 3.6489) (-1.3651, 3.6505) (-1.3657, 3.6967) (-1.362, 3.7769) (-1.3649, 3.8524) (-1.367, 3.9088) (-1.3751, 3.9479) (-1.3714, 3.9993) (-1.3701, 4.0175) (-1.3754, 4.0652) (-1.3096, 4.0975) (-1.2377, 4.1328) (-1.2058, 4.0937) (-1.195, 4.0864) (-1.1814, 4.0773) (-1.1803, 4.076) (-1.1783, 4.0748) knots 0.954762 0.954762 0.954762 0.954762 0.954962 0.954962 0.954962 0.96088 0.96088 0.96088 0.965295 0.965295 0.965295 0.966859 0.966859 0.966859 0.968566 0.968566 0.968566 0.970711 0.970711 0.970711 0.970711
  spline S8 degree 3 poles (-1.1783, 4.0748) (-1.1765, 4.0743) (-1.1692, 4.0734) (-1.1532, 4.0723) (-1.1185, 4.07) (-1.0855, 4.0632) (-1.0714, 4.0662) (-1.0634, 4.0679) (-1.0453, 4.076) (-1.0187, 4.0876) (-1.0023, 4.0947) (-0.9908, 4.1239) (-0.9161, 4.0968) (-0.8648, 4.0781) (-0.844, 4.0106) (-0.8447, 3.9886) (-0.8451, 3.9749) (-0.8471, 3.9668) (-0.8481, 3.9619) knots 0.972261 0.972261 0.972261 0.972261 0.974755 0.974755 0.974755 0.980187 0.980187 0.980187 0.983279 0.983279 0.983279 0.985179 0.985179 0.985179 0.986486 0.986486 0.986486 0.987304 0.987304 0.987304 0.987304
  spline S9 degree 3 poles (-0.8481, 3.9619) (-0.8469, 3.9546) (-0.8451, 3.9422) (-0.8442, 3.9291) knots 0.991152 0.991152 0.991152 0.991152 0.992517 0.992517 0.992517 0.992517
  point P0 (-0.7897, 3.8423)
  point P1 (-0.6129, 3.9328)
  point P2 (-0.3195, 4.1014)
  point P3 (-0.0097, 4.2755)
  point P4 (0.3426, 4.4757)
  point P5 (0.6099, 4.6251)
  point P6 (0.9, 4.8)
  point P7 (1.2707, 5.0131)
  point P8 (1.4284, 5.1036)
  point P9 (1.55, 5.15)
  point P10 (1.6504, 5.1721)
  point P11 (1.9452, 5.179)
  point P12 (2.2344, 5.1872)
  point P13 (2.4648, 5.1899)
  point P14 (2.643, 5.168)
  point P15 (2.75, 5.1)
  point P16 (2.8376, 4.9733)
  point P17 (2.9281, 4.7951)
  point P18 (2.9884, 4.6868)
  point P19 (3.1104, 4.4647)
  point P20 (3.2325, 4.244)
  point P21 (3.25, 4.2)
  point P22 (3.2695, 4.1097)
  point P23 (3.2832, 4)
  point P24 (3.2215, 3.8588)
  point P25 (2.9857, 3.4585)
  point P26 (2.7801, 3.1075)
  point P27 (2.6868, 2.9252)
  point P28 (2.5539, 2.7292)
  point P29 (2.3345, 2.6058)
  point P30 (1.9274, 2.5701)
  point P31 (1.5065, 2.5756)
  point P32 (1.2, 2.55)
  point P33 (0.9664, 2.5057)
  point P34 (0.8, 2.45)
  point P35 (0.6182, 2.2329)
  point P36 (0.45, 2.05)
  point P37 (0.3234, 1.7517)
  point P38 (0.2796, 1.5982)
  point P39 (0.25, 1.45)
  point P40 (0.2878, 1.2459)
  point P41 (0.418, 1.0594)
  point P42 (0.4537, 1.0334)
  point P43 (0.4674, 1.0169)
  point P44 (0.45, 1)
  point P45 (0.42, 1)
  point P46 (0.2875, 0.966)
  point P47 (0.0939, 0.8386)
  point P48 (-0.0168, 0.7247)
  point P49 (-0.14, 0.48)
  point P50 (-0.22, 0.27)
  point P51 (-0.28, 0.07)
  point P52 (-0.33, -0.08)
  point P53 (-0.3938, -0.275)
  point P54 (-0.4255, -0.3855)
  point P55 (-0.51, -0.69)
  point P56 (-0.5866, -1.0357)
  point P57 (-0.6161, -1.1144)
  point P58 (-0.65, -1.3)
  point P59 (-0.6811, -1.5848)
  point P60 (-0.6811, -1.8524)
  point P61 (-0.64, -2.08)
  point P62 (-0.49, -2.24)
  point P63 (-0.29, -2.3)
  point P64 (-0.18, -2.3)
  point P65 (-0.02, -2.3)
  point P66 (0.5, -2.3)
  point P67 (0.63, -2.3)
  point P68 (1.28, -2.3)
  point P69 (1.99, -2.3)
  point P70 (2.17, -2.3)
  point P71 (2.46, -2.29)
  point P72 (2.6, -2.29)
  point P73 (2.63, -2.29)
  point P74 (2.68, -2.3)
  point P75 (2.72, -2.31)
  point P76 (2.77, -2.37)
  point P77 (2.8, -2.43)
  point P78 (2.78, -2.57)
  point P79 (2.73, -2.74)
  point P80 (2.6, -3.24)
  point P81 (2.52, -3.57)
  point P82 (2.5, -3.65)
  point P83 (2.46, -3.72)
  point P84 (2.43, -3.76)
  point P85 (2.42, -3.71)
  point P86 (2.42, -3.63)
  point P87 (2.41, -3.59)
  point P88 (2.33, -3.59)
  point P89 (2.26, -3.58)
  point P90 (2.21, -3.43)
  point P91 (2.19, -3.1)
  point P92 (2.19, -3.03)
  point P93 (2.18, -2.97)
  point P94 (2.01, -2.95)
  point P95 (1.92, -2.95)
  point P96 (1.07, -2.95)
  point P97 (0.3354, -2.9829)
  point P98 (-1.5187, -2.9829)
  point P99 (-2.15, -3)
  point P100 (-2.45, -3)
  point P101 (-2.5, -3.05)
  point P102 (-2.55, -3.3)
  point P103 (-2.5704, -3.5002)
  point P104 (-2.7791, -3.6036)
  point P105 (-2.8056, -3.6226)
  point P106 (-2.81, -3.71)
  point P107 (-2.81, -3.77)
  point P108 (-2.82, -3.79)
  point P109 (-2.9543, -3.7968)
  point P110 (-3.02, -3.77)
  point P111 (-3.06, -3.69)
  point P112 (-3.0573, -3.5546)
  point P113 (-3.01, -3.44)
  point P114 (-2.96, -3.26)
  point P115 (-2.9025, -3.0455)
  point P116 (-2.8553, -2.8671)
  point P117 (-2.808, -2.7308)
  point P118 (-2.75, -2.6)
  point P119 (-2.7287, -2.479)
  point P120 (-2.6745, -2.3622)
  point P121 (-2.5896, -2.3246)
  point P122 (-2.4588, -2.2634)
  point P123 (-2.3545, -2.1201)
  point P124 (-2.3, -1.9)
  point P125 (-2.2237, -1.6471)
  point P126 (-2.1709, -1.4162)
  point P127 (-2.0958, -1.1686)
  point P128 (-2.0165, -0.8514)
  point P129 (-1.9706, -0.6998)
  point P130 (-1.8871, -0.4091)
  point P131 (-1.7508, -0.0348)
  point P132 (-1.65, 0.25)
  point P133 (-1.5616, 0.5077)
  point P134 (-1.4656, 0.8374)
  point P135 (-1.4, 1.1)
  point P136 (-1.3432, 1.27)
  point P137 (-1.3334, 1.4801)
  point P138 (-1.3974, 1.7277)
  point P139 (-1.5435, 1.9364)
  point P140 (-1.6687, 2.0504)
  point P141 (-1.7688, 2.1742)
  point P142 (-1.7981, 2.3314)
  point P143 (-1.8, 2.7)
  point P144 (-1.7994, 3.0339)
  point P145 (-1.7549, 3.2204)
  point P146 (-1.6395, 3.3636)
  point P147 (-1.4628, 3.4749)
  point P148 (-1.3223, 3.5514)
  point P149 (-1.268, 3.5973)
  point P150 (-1.2625, 3.6377)
  point P151 (-1.2625, 3.8547)
  point P152 (-1.2666, 4.0035)
  point P153 (-1.25, 4)
  point P154 (-1.204, 3.9757)
  point P155 (-1.1275, 3.9674)
  point P156 (-1.0302, 3.9716)
  point P157 (-0.95, 4)
  point P158 (-0.95, 3.9757)
  point P159 (-0.95, 3.95)
  point P160 (-0.95, 3.838)
  dimension "d2" = -0.1024
extrude "Extrude1" add sketch "Sketch2" along normal blind 0.3
